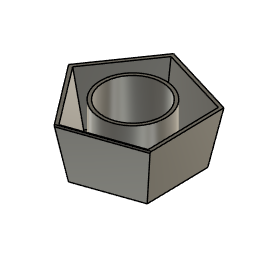
10409김태균_스케치 (Autodesk Fusion 360 design; units mm, degrees)
Autodesk Fusion 360 part; units mm, degrees
sketch "스케치1" plane through (0, 0, 0) normal (0, 0, 1) x (1, 0, 0)
  line L0 (-15, 6) -> (-22, -7)
  line L1 (-22, -7) -> (-9, -9)
  line L2 (-9, -9) -> (-3, 0)
  line L3 (-3, 0) -> (-12, 7)
  line L4 (3, 5) -> (3, -9.4098)
  line L5 (3, -9.4098) -> (20.2982, -14.6076)
  line L6 (20.2982, -14.6076) -> (26.171, 4.9371)
  line L7 (26.171, 4.9371) -> (7.7071, 8.424)
  line L8 (42.6307, 4.9371) -> (42, -15)
  line L9 (42, -15) -> (67.9355, -17.567)
  line L10 (67.9355, -17.567) -> (65.6256, 5.8006)
  line L11 (65.6256, 5.8006) -> (42.6307, 4.9371)
  line L12 (78.9292, 2.5635) -> (78.4348, -13.0662)
  line L13 (78.4348, -13.0662) -> (106, -18)
  arc A0 (106, -18) -> (78.9292, 2.5635) centre (112.5801, 18.7627) ccw
  line L14 (-78.1892, -7.301) -> (-40, -7.301)
  line L15 (-40, -7.301) -> (-40, 37.2455)
  arc A1 (-40, 37.2455) -> (-75, 40) centre (-57.6084, 37.2455) ccw
  line L16 (-75, 40) -> (-75, -7.301)
  line L17 (-75, -25) -> (-35, -25)
  line L18 (-35, -25) -> (-35, -65)
  line L19 (-35, -65) -> (-75, -65)
  line L20 (-75, -65) -> (-75, -25)
  line L21 (20, -31.5) -> (70, -31.5)
  line L22 (70, -31.5) -> (70, -81.5)
  line L23 (70, -81.5) -> (20, -81.5)
  line L24 (20, -81.5) -> (20, -31.5)
  line L25 (100.3878, -38.2853, -0.4734) -> (160.3878, -38.2853, -0.4734)
  line L26 (160.3878, -38.2853, -0.4734) -> (160.3878, -98.2853, -0.4734)
  line L27 (160.3878, -98.2853, -0.4734) -> (100.3878, -98.2853, -0.4734)
  line L28 (100.3878, -98.2853, -0.4734) -> (100.3878, -38.2853, -0.4734)
  line L29 (100.3878, -98.2853, -0.4734) -> (160.3878, -38.2853, -0.4734) construction
  line L30 (100.3878, -38.2853, -0.4734) -> (160.3878, -98.2853, -0.4734) construction
  line L31 (221.7769, -77.0241) -> (180.313, -77.0241)
  line L32 (180.313, -77.0241) -> (180.313, -31.5347)
  line L33 (180.313, -31.5347) -> (221.7769, -31.5347)
  line L34 (221.7769, -31.5347) -> (221.7769, -77.0241)
  line L35 (221.7769, -77.0241) -> (180.313, -31.5347) construction
  line L36 (180.313, -77.0241) -> (221.7769, -31.5347) construction
  circle A2 centre (-30, -160) radius 25.461
  circle A3 centre (27.6815, -165.0053) radius 31.7614
  circle A4 centre (125.6318, -141.5124) radius 31.894
  circle A5 centre (125.6318, -141.5124) radius 31.894
  circle A6 centre (157.3931, -144.4186) radius 36.4671
  circle A7 centre (190.6677, -144.4186) radius 5.5401
  circle A8 centre (152.4397, -176.5897) radius 12.8987
  circle A9 centre (125.6318, -192.8529) radius 43.2366
  circle A10 centre (125.6318, -173.4064) radius 27.8792
  line L37 (-174.3672, -75.4378) -> (-188.8141, -19.5395)
  line L38 (-188.8141, -19.5395) -> (-244.4468, -4.1017)
  line L39 (-244.4468, -4.1017) -> (-285.6328, -44.5622)
  line L40 (-285.6328, -44.5622) -> (-271.1859, -100.4605)
  line L41 (-271.1859, -100.4605) -> (-215.5532, -115.8983)
  line L42 (-215.5532, -115.8983) -> (-174.3672, -75.4378)
  line L43 (-160.849, -213.9216) -> (-162.0762, -155.1559)
  line L44 (-162.0762, -155.1559) -> (-218.345, -138.1635)
  line L45 (-218.345, -138.1635) -> (-251.8938, -186.4273)
  line L46 (-251.8938, -186.4273) -> (-216.3593, -233.2484)
  line L47 (-216.3593, -233.2484) -> (-160.849, -213.9216)
  point P0 (201.045, -54.2794)
  point P1 (-230, -60)
  point P2 (-201.9047, -185.3833)
  dimension "d1" = 40
  dimension "d2" = 40
  dimension "d3" = 50
  dimension "d4" = 50
  dimension "d5" = 50
  dimension "d6" = 60
  dimension "d7" = 60
  dimension "d8" = 60
  dimension "d9" = 50
  dimension "d10" = 50
  constraint vertical L4
  constraint perpendicular L5 L6
  constraint parallel L8 L12
  constraint tangent L13 A0
  constraint horizontal L14
  constraint perpendicular L14 L15
  constraint tangent L15 A1
  constraint coincident L14 L16.end
  constraint perpendicular L14 L16
  constraint horizontal L17
  constraint vertical L18
  constraint horizontal L19
  constraint vertical L20
  constraint horizontal L21
  constraint vertical L22
  constraint horizontal L23
  constraint vertical L24
  constraint horizontal L31
  constraint perpendicular L31 L32
  constraint parallel L31 L33
  constraint parallel L32 L34
  constraint coincident L35 P0
  constraint coincident L36 P0
  constraint concentric A4 A5
  constraint coincident A4 A6.centre
  constraint coincident A5 A10.centre
  measures "d1" distance of L18.end L19.end
  measures "d2" distance of L17.end L18.end
  measures "d3" distance of L21.start L23.end
  measures "d4" distance of L22.end L23.end
  measures "d5" distance of L22.end L23.end
  measures "d9" distance of P1 L42
  measures "d10" distance of L43.start P2
extrude "돌출1" add sketch "스케치1" along normal blind 50 draft 10 contours L43 L44 L45 L46 L47
sketch "스케치2" plane through (0, 0, 50) normal (0, 0, 1) x (-1, 0, 0)
  circle A0 centre (203.6154, 184.7621) radius 27.8241
extrude "돌출2" cut sketch "스케치2" against normal blind 50
shell "쉘1" thickness 3 removed faces 1 at (-160.3626, -184.4905, 50)
fillet "필렛1" radius 1 2 edges at (-185.7053, -231.9111, 50) (-186.7069, -229.0342, 50)
